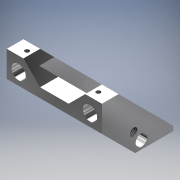
# Autodesk Inventor part: led halter 2
Saved by Autodesk Inventor 2017 (Build 210142000, 142)
## iProperties
Part Number: led halter 2
Material: Aluminium 6061
Document SubType Name: Modeling
Designer: David Merges
Density: 2.7 g/cm^3
Appearance: Aluminium - flach
Author: David Merges
Autodesk Inventor part; units mm, degrees
ref_plane "YZ Plane" through (0, 0, 0) normal (1, 0, 0) x (0, 1, 0)
ref_plane "XZ Plane" through (0, 0, 0) normal (0, 1, 0) x (-1, 0, 0)
ref_plane "XY Plane" through (0, 0, 0) normal (0, 0, 1) x (1, 0, 0)
sketch "Skizze1" plane through (0, 0, 0) normal (0, 1, 0) x (-1, 0, 0)
  line L0 (20, 20) -> (-20, 20)
  line L1 (-20, 20) -> (-20, -20)
  line L2 (-20, -20) -> (20, -20)
  line L3 (20, -20) -> (20, 20)
  line L4 (20, -20) -> (-20, 20) construction
  point P0 (0, 0)
  point P1 (0, 0)
  dimension "d0" = 40
  dimension "d1" = 40
  constraints: 10 end point, 2 parallel, 1 coincident, 1 horizontal, 1 midpoint, 1 perpendicular
  measures "d0" distance of L2.end L1.end
  measures "d1" distance of L1.end L0.end
extrude "Extrusion1" add sketch "Skizze1" along normal mid plane 10
sketch "Skizze2" plane through (0, -5, 0) normal (0, -1, 0) x (1, 0, 0)
  line L0 (-15, 15) -> (15, 15) construction
  line L1 (15, 15) -> (15, -15) construction
  line L2 (15, -15) -> (-15, -15) construction
  line L3 (-15, -15) -> (-15, 15) construction
  line L4 (15, -15) -> (-15, 15) construction
  point P0 (0, 0)
  dimension "d4" = 30
  dimension "d5" = 30
  constraints: 10 end point, 2 midpoint, 2 parallel, 1 horizontal, 1 perpendicular
  measures "d4" distance of L1.end L2.end
  measures "d5" distance of L0.end L1.end
hole "Bohrung1" at (15, -5, -15) at (15, -5, 15) at (-15, -5, 15) at (-15, -5, -15) direction (0, 1, 0) diameter 6 end through all
sketch "Skizze12" plane through (-20, 5, 20) normal (0, 0, 1) x (1, 0, 0)
  line L0 (40, -10) -> (40, 0) projected
  line L1 (0, 0) -> (40, 0) projected
  line L2 (0, 0) -> (0, -10) projected
  line L3 (40, -10) -> (0, -10) projected
  point P0 (20, -5)
extrude "Extrusion8" cut sketch "Skizze12" against normal blind 29
sketch "Skizze13" plane through (20, 5, -20) normal (0, 0, -1) x (-1, 0, 0)
  line L0 (40, -10) -> (40, 0) projected
  line L1 (0, 0) -> (40, 0) projected
  line L2 (0, -10) -> (0, 0) projected
  line L3 (40, -10) -> (0, -10) projected
  point P0 (20, -5)
extrude "Extrusion9" add sketch "Skizze13" along normal blind 20
sketch "Skizze14" plane through (0, 5, 0) normal (0, 1, 0) x (1, 0, 0)
  line L0 (-20, 9) -> (20, 9) projected
  line L1 (20, 9) -> (20, 40) projected
  line L2 (-20, 40) -> (20, 40) projected
  line L3 (-20, 9) -> (-20, 40) projected
  circle A0 centre (-15, 15) radius 3 projected
  circle A1 centre (15, 15) radius 3 projected
  point P0 (0, 0)
extrude "Extrusion10" add sketch "Skizze14" along normal blind 20
sketch "Skizze16" plane through (0, -5, 0) normal (0, -1, 0) x (1, 0, 0)
  circle A0 centre (0, 0) radius 15
  line L0 (20, -9) -> (-20, -9) projected
  line L1 (-20, -9) -> (-20, -40) projected
  line L2 (20, -40) -> (-20, -40) projected
  line L3 (20, -9) -> (20, -40) projected
  circle A1 centre (15, -15) radius 3 projected
  circle A2 centre (-15, -15) radius 3 projected
  line L4 (20, -9) -> (-20, -9) projected
  line L5 (-13, -9) -> (-6, -16)
  line L6 (0, -22) -> (6, -16) construction
  line L7 (-6, -16) -> (6, -16)
  line L8 (0, -9) -> (0, -22) construction
  line L9 (-6, -16) -> (0, -22) construction
  line L10 (6, -16) -> (13, -9)
  line L11 (13, -9) -> (-13, -9)
  dimension "d68" = 30
  dimension "d69" = 45
  dimension "d70" = 7
  dimension "d71" = 7
  constraints: 14 end point, 5 perpendicular, 2 point on line, 1 centre point, 1 coincident, 1 collinear, 1 horizontal, 1 midpoint
  measures "d68" diameter of A0
  measures "d69" angle of L0 L6
  measures "d70" distance between parallel lines of L0 L7
  measures "d71" distance of L0.end L5.start
extrude "Extrusion12" cut sketch "Skizze16" against normal through all contours L0 A0 | A0 L0 L10 L7 L5 picked at (-3.2037, -9.8388)
sketch "Skizze17" plane through (20, -5, -9) normal (1, 0, 0) x (0, 0, -1)
  line L0 (7, 0) -> (7, 30) construction
  line L1 (7, 0) -> (7, 30) projected
  line L2 (0, 30) -> (0, 0) projected
  line L3 (0, 0) -> (31, 0) construction
  line L4 (31, 0) -> (31, 30) construction
  line L5 (0, 30) -> (31, 30) projected
  line L6 (23, 30) -> (0, 7)
  line L7 (0, 30) -> (0, 0) projected
  line L8 (7, 14) -> (23, 30)
  line L9 (0, 30) -> (31, 30) projected
  line L10 (23, 30) -> (0, 30)
  line L11 (0, 30) -> (0, 7)
  point P0 (-9, 5)
  dimension "d74" = 45
  dimension "d78" = 7
  constraints: 8 end point, 4 point on line, 2 collinear, 1 perpendicular
  measures "d74" angle of L5 L6
  measures "d78" distance of L2.end L6.end
extrude "Extrusion13" cut sketch "Skizze17" against normal through all
sketch "Skizze18" plane through (20, 5, -40) normal (0, 0, -1) x (-1, 0, 0)
  line L0 (40, -10) -> (40, 20) projected
  line L1 (0, 20) -> (40, 20) projected
  line L2 (0, -10) -> (0, 20) projected
  line L3 (0, -10) -> (40, -10) projected
  point P0 (20, -5)
extrude "Extrusion14" cut sketch "Skizze18" against normal blind 6
sketch "Skizze19" plane through (20, -5, -9) normal (1, 0, 0) x (0, 0, -1)
  line L0 (25, 0) -> (25, 30) projected
  line L1 (23, 30) -> (25, 30) projected
  line L2 (23, 30) -> (0, 7) projected
  line L3 (0, 7) -> (0, 0) projected
  line L4 (0, 0) -> (25, 0) projected
  line L5 (11, 0) -> (25, 14)
  line L6 (25, 0) -> (25, 30) projected
  point P0 (-9, 5)
  dimension "d81" = 45
  dimension "d82" = 14
  constraints: 2 end point, 2 point on line
  measures "d81" angle of L4 L5
  measures "d82" distance from line of L5.start L0
extrude "Extrusion15" cut sketch "Skizze19" against normal through all contours L4 L5 L0
sketch "Skizze21" plane through (-20, 5, -9) normal (0, 0, 1) x (1, 0, 0)
  circle A0 centre (5, 3) radius 3 projected
  line L0 (8, -10) -> (2, -10) projected
  circle A1 centre (35, 3) radius 3 projected
  line L1 (38, -10) -> (32, -10) projected
  line L2 (0, -3) -> (0, 20) construction
  line L3 (7, -3) -> (0, -3) construction
  line L4 (14, 4) -> (7, -3) construction
  line L5 (26, 4) -> (14, 4) construction
  line L6 (33, -3) -> (26, 4) construction
  line L7 (40, -3) -> (33, -3) construction
  line L8 (40, 20) -> (40, -3) construction
  line L9 (0, 20) -> (40, 20) construction
  circle A2 centre (35, 3) radius 3 construction
  circle A3 centre (5, 3) radius 3 construction
  line L10 (5, -10) -> (5, -3) construction
  line L11 (40, -10) -> (33, -10) construction
  line L12 (35, -10) -> (35, -3) construction
  line L13 (40, -3) -> (33, -3) construction
  point P0 (20, -5)
  point P1 (35, -6.5)
  point P2 (5, -6.5)
  constraints: 4 end point, 3 midpoint, 3 point on line, 1 perpendicular, 1 vertical
hole "Bohrung5" at (15, -1.5, -9) at (-15, -1.5, -9) direction (0, 0, -1) diameter 1.813 depth 7.2 tip angle 118 thread size "M2.3x0.45" class "6H" standard "ISO Metric profile"
sketch "Skizze23" plane through (-20, 25, -32) normal (0, 0.7071068, 0.7071068) x (1, 0, 0)
  line L0 (0, -32.5269) -> (0, 0) projected
  line L1 (7, -32.5269) -> (0, -32.5269) projected
  line L2 (14, -22.6274) -> (7, -32.5269) projected
  line L3 (26, -22.6274) -> (14, -22.6274) projected
  line L4 (33, -32.5269) -> (26, -22.6274) projected
  line L5 (40, -32.5269) -> (33, -32.5269) projected
  line L6 (40, 0) -> (40, -32.5269) projected
  line L7 (0, 0) -> (40, 0) projected
  ellipse E0 centre (35, -24.0416) end of major axis (35, -28.2843) minor radius 3 projected
  ellipse E1 centre (5, -24.0416) end of major axis (5, -28.2843) minor radius 3 projected
  line L8 (30, 0) -> (30, -16.6274)
  line L9 (0, 0) -> (40, 0) projected
  line L10 (10, 0) -> (10, -16.6274)
  line L11 (30, 0) -> (10, 0) construction
  line L12 (24, -22.6274) -> (16, -22.6274)
  arc A0 (24, -22.6274) -> (30, -16.6274) centre (24, -16.6274) ccw
  arc A1 (10, -16.6274) -> (16, -22.6274) centre (16, -16.6274) ccw
  line L13 (40, 1.4142) -> (0, 1.4142) construction
  line L14 (0, 1.4142) -> (0, 0) projected
  line L15 (0, 0) -> (40, 0) projected
  line L16 (40, 0) -> (40, 1.4142) projected
  line L17 (30, 0) -> (30, 1.4142)
  line L18 (40, 1.4142) -> (0, 1.4142) construction
  line L19 (10, 0) -> (10, 1.4142)
  line L20 (30, 1.4142) -> (10, 1.4142)
  line L21 (30, -16.6274) -> (30, -28.2843)
  line L22 (10, -16.6274) -> (10, -28.2843)
  line L23 (14, -22.6274) -> (7, -32.5269) projected
  line L24 (30, -28.2843) -> (10, -28.2843)
  line L25 (33, -32.5269) -> (26, -22.6274) projected
  line L26 (26, -32.5269) -> (26, -22.6274) projected
  line L27 (33, -37.4767) -> (26, -32.5269) projected
  line L28 (33, -32.5269) -> (33, -37.4767) projected
  line L29 (14, -22.6274) -> (7, -32.5269) projected
  line L30 (7, -37.4767) -> (7, -32.5269) projected
  line L31 (14, -32.5269) -> (7, -37.4767) projected
  line L32 (14, -32.5269) -> (14, -22.6274) projected
  line L33 (30, -28.2843) -> (30, -35.3553)
  line L34 (33, -37.4767) -> (26, -32.5269) projected
  line L35 (10, -28.2843) -> (10, -35.3553)
  line L36 (30, -35.3553) -> (10, -35.3553)
  point P0 (20, -40.3051)
  point P1 (20, 0)
  dimension "d99" = 20
  dimension "d100" = 6
  constraints: 26 end point, 10 point on line, 4 point on circle, 4 tangent, 3 perpendicular, 3 vertical, 2 centre point, 2 collinear, 2 horizontal, 2 midpoint, 2 parallel, 1 equal radius, 2 other
  measures "d99" distance between parallel lines of L10 L8
  measures "d100" radius of A0
extrude "Extrusion16" cut sketch "Skizze23" against normal blind 4.5 contours L19 L20 L17 L7 | L7 L8 A0 L3 A1 L10 | L22 A1 L3 L2 | L2 L32 L24 | L24 L32 L31 L35 | L3 L26 L24 L32 | L24 L26 L27 L36 L31 L32 | L21 L4 L3 A0 | L26 L4 L24 | L24 L33 L27 L26
sketch "Skizze24" plane through (20, -5, -9) normal (1, 0, 0) x (0, 0, -1)
  line L0 (11, 0) -> (25, 14) projected
  line L1 (25, 14) -> (25, 30) projected
  line L2 (23, 30) -> (25, 30) projected
  line L3 (23, 30) -> (0, 7) projected
  line L4 (0, 7) -> (0, 0) projected
  line L5 (0, 0) -> (11, 0) projected
  line L6 (3, 3.636) -> (25, 25.636) projected
  line L7 (7, 7.636) -> (3, 3.636) projected
  line L8 (3, 3.636) -> (7, 7.636) projected
  line L9 (25, 25.636) -> (3, 3.636) projected
  line L10 (9, 16) -> (9, 0) projected
  line L11 (9, 16) -> (9, 0) construction
  line L12 (9, 5.3934) -> (25, 21.3934) construction
  line L13 (25, 30) -> (25, 14) construction
  line L14 (17, 13.3934) -> (17, 17.636) construction
  line L15 (3, 3.636) -> (25, 25.636) construction
  line L16 (17, 13.3934) -> (17, 6) construction
  line L17 (11, 0) -> (25, 14) construction
  point P0 (-9, 5)
  dimension "d103" = 3
  constraints: 6 end point, 5 point on line, 1 coincident, 1 midpoint, 1 parallel, 1 vertical
  measures "d103" distance between parallel lines of L6 L12
hole "Bohrung7" at (20, 8.3934, -26) direction (-1, 0, 0) diameter 3.242 end through all thread size "M4x0.7" class "6H" standard "ISO Metric profile"
thread "Gewinde1" size "M4x0.7" class "6H" standard "ISO Metric profile" length 10
thread "Gewinde2" size "M4x0.7" class "6H" standard "ANSI Metric M Profile" length 10
sketch "Skizze25" plane through (20, -5, -9) normal (1, 0, 0) x (0, 0, -1)
  circle A0 centre (17, 13.3934) radius 1.621 projected
  line L0 (11, 0) -> (25, 14) projected
  line L1 (25, 14) -> (25, 30) projected
  line L2 (23, 30) -> (25, 30) projected
  line L3 (23, 30) -> (0, 7) projected
  line L4 (0, 7) -> (0, 0) projected
  line L5 (0, 0) -> (11, 0) projected
  circle A1 centre (21.5, 16.7) radius 2.5
  line L6 (25, 25.636) -> (3, 3.636) projected
  point P0 (-9, 5)
  dimension "d115" = 5
  dimension "d116" = 3.5
  dimension "d117" = 2.7
  constraints: 1 centre point
  measures "d115" diameter of A1
  measures "d116" distance from line of A1.centre L1
  measures "d117" vertical distance of A1.centre L0.end
extrude "Extrusion17" cut sketch "Skizze25" against normal blind 5 contours A1
